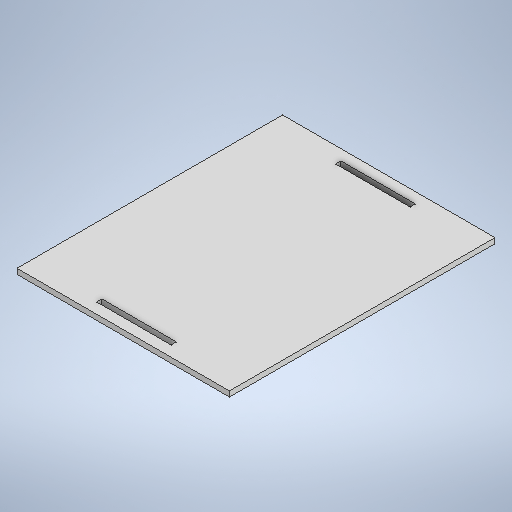
# Autodesk Inventor part: top
Saved by Autodesk Inventor 2025.3 (Build 293356030, 356C)
## iProperties
Created: 2026-06-26
Part Number: top
Material: Generic
Document SubType Name: Modeling
Designer: user
Density: 1 g/cm^3
Appearance: Default
Author: user
Autodesk Inventor part; units mm, degrees
ref_plane "YZ Plane" through (0, 0, 0) normal (1, 0, 0) x (0, 1, 0)
ref_plane "XZ Plane" through (0, 0, 0) normal (0, 1, 0) x (-1, 0, 0)
ref_plane "XY Plane" through (0, 0, 0) normal (0, 0, 1) x (1, 0, 0)
sketch "Sketch1" plane through (0, 0, 0) normal (0, 1, 0) x (-1, 0, 0)
  line L0 (0, 0) -> (-200, 0)
  line L1 (-200, 0) -> (-200, -250)
  line L2 (-200, -250) -> (0, -250)
  line L3 (0, -250) -> (0, 0)
  line L4 (-65, -10) -> (-135, -10)
  line L5 (-135, -10) -> (-135, -15)
  line L6 (-135, -15) -> (-65, -15)
  line L7 (-65, -15) -> (-65, -10)
  line L8 (-200, -125) -> (0, -125) construction
  line L9 (-65, -240) -> (-135, -240)
  line L10 (-135, -240) -> (-135, -235)
  line L11 (-135, -235) -> (-65, -235)
  line L12 (-65, -235) -> (-65, -240)
  line L13 (-200, -235) -> (-200, -35)
  dimension "d0" = 200
  dimension "d2" = 70
  dimension "d3" = 5
  dimension "d11" = 10
  dimension "d12" = 230
  constraints: 28 end point, 4 parallel, 4 symmetric about line, 2 horizontal, 2 midpoint, 2 perpendicular, 1 point on line
  measures "d0" distance of L2.end L1.end
  measures "d2" distance of L6.end L5.end
  measures "d3" distance of L5.end L4.end
  measures "d11" distance between parallel lines of L0 L4
  measures "d12" distance between parallel lines of L4 L9
extrude "Extrusion1" add sketch "Sketch1" along normal blind 5
body "Solid1"
